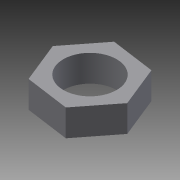
# Autodesk Inventor part: 8mm-thin-nut
Saved by Autodesk Inventor 2014 (Build 180170000, 170)
## iProperties
Created: 2013-11-06
Part Number: 8mm-thin-nut
Material: Generic
Document SubType Name: Modeling
Designer: stephen
Density: 1 g/cm^3
Appearance: Default
Author: stephen
Autodesk Inventor part; units mm, degrees
ref_plane "YZ Plane" through (0, 0, 0) normal (1, 0, 0) x (0, 1, 0)
ref_plane "XZ Plane" through (0, 0, 0) normal (0, 1, 0) x (-1, 0, 0)
ref_plane "XY Plane" through (0, 0, 0) normal (0, 0, 1) x (1, 0, 0)
sketch "Sketch1" plane through (0, 0, 0) normal (0, 1, 0) x (-1, 0, 0)
  line L0 (-17.9573, -28.8171) -> (-24.4573, -27.9026)
  line L1 (-24.4573, -27.9026) -> (-26.9153, -21.8162)
  line L2 (-26.9153, -21.8162) -> (-22.8733, -16.6443)
  line L3 (-22.8733, -16.6443) -> (-16.3733, -17.5588)
  line L4 (-16.3733, -17.5588) -> (-13.9153, -23.6453)
  line L5 (-13.9153, -23.6453) -> (-17.9573, -28.8171)
  circle A0 centre (-20.4153, -22.7307) radius 4
  dimension "d12" = 13
  dimension "d13" = 8
  constraints: 12 end point, 1 centre point, 1 coincident, 13 other
  measures "d12" horizontal distance of L4.end L1.end
  measures "d13" diameter of A0
extrude "Extrusion1" add sketch "Sketch1" along normal blind 4
body "Solid1"
